# Autodesk Inventor part: Kettenrad der Rollenkette1
Saved by Autodesk Inventor 2016 (Build 200138000, 138)
## iProperties
Created: 2017-12-11
Part Number: Kettenrad der Rollenkette1
Material: Steel
Document SubType Name: Modeling
Designer: Dominik
Density: 1 g/cm^3
Appearance: Steel
CustomPartVersion: 1
Author: Dominik
Autodesk Inventor part; units mm, degrees
ref_plane "YZ Plane" through (0, 0, 0) normal (1, 0, 0) x (0, 1, 0)
ref_plane "XZ Plane" through (0, 0, 0) normal (0, 1, 0) x (-1, 0, 0)
sketch "Theoretisches Zahnprofil" plane through (0, 0, 0) normal (0, 0, 1) x (1, 0, 0)
  circle A0 centre (0, 0) radius 24.3021 construction
  line L0 (0, 0) -> (0, 24.3021) construction
  line L1 (0, 0) -> (7.8909, 22.9854) construction
  circle A1 centre (0, 0) radius 26.3707
  arc A2 (-1.9854, 22.7421) -> (1.9854, 22.7421) centre (0, 24.3021) ccw
  line L2 (0, 24.3021) -> (7.8909, 22.9854) construction
  line L3 (0, 24.3021) -> (3.1452, 26.7735) construction
  line L4 (3.1452, 26.7735) -> (-2.8564, 24.2129) construction
  arc A3 (3.9692, 26.0703) -> (3.0961, 24.7748) centre (6.9045, 23.15) ccw
  arc A4 (-3.0961, 24.7748) -> (-3.9692, 26.0703) centre (-6.9045, 23.15) ccw
  line L5 (-6.9045, 23.15) -> (-3.0961, 24.7748) construction
  arc A5 (-2.8564, 24.2129) -> (-1.9854, 22.7421) centre (3.1452, 26.7735) ccw
  line L6 (-2.8564, 24.2129) -> (-3.0961, 24.7748)
  arc A6 (1.9854, 22.7421) -> (2.8564, 24.2129) centre (-3.1452, 26.7735) ccw
  line L7 (3.0961, 24.7748) -> (2.8564, 24.2129)
  line L8 (0, 0) -> (4.3405, 26.011) construction
  point P0 (3.9454, 23.6438)
  dimension "d0" = 48.6043
  dimension "d2" = 18.947
  dimension "d3" = 2.525
  dimension "d10" = 128.158
  dimension "d11" = 15.053
  dimension "d12" = 4
  dimension "d13" = 6.525
  dimension "d14" = 7
  dimension "d23" = 2.4
  constraints: 18 end point, 15 point on circle, 7 centre point, 3 coincident, 3 point on line, 3 symmetric about line, 3 tangent, 1 equal radius, 1 midpoint, 1 parallel, 1 vertical, 1 other
  measures "d0" diameter of A0
  measures "d2" angle of L1 L0
  measures "d3" radius of A2
  measures "d10" angle of L3 L0
  measures "d11" angle of L4 L3
  measures "d12" distance of L2.start L3.end
  measures "d13" distance of L3.end L4.end
  measures "d14" distance of A3.centre L0.end
  measures "d23" distance from line of L8.end L2
sketch "Zahnprofil" plane through (0, 0, 0) normal (0, 0, 1) x (1, 0, 0)
  arc A0 (-2.335, 23.3412) -> (2.335, 23.3412) centre (0, 24.3021) ccw
  arc A1 (3.8891, 26.0823) -> (2.335, 23.3412) centre (13.9869, 18.5462) ccw
  arc A2 (-2.335, 23.3412) -> (-3.8891, 26.0823) centre (-13.9869, 18.5462) ccw
  line L0 (0, 0) -> (0, 24.3021) construction
  line L1 (0, 24.3021) -> (2.335, 23.3412) construction
  line L2 (0, 24.3021) -> (-2.335, 23.3412) construction
  circle A3 centre (0, 0) radius 26.3707 projected
  dimension "d44" = 135.263
  dimension "d45" = 12.6
  dimension "d46" = 2.525
  constraints: 9 point on circle, 6 end point, 3 centre point, 2 tangent, 1 coincident, 1 equal radius, 1 vertical, 1 other
  measures "d44" angle of L2 L1
  measures "d45" radius of A1
  measures "d46" radius of A0
sketch "Schnittprofil" plane through (0, 0, 0) normal (1, 0, 0) x (0, 1, 0)
  line L0 (26.3707, 0) -> (-26.3707, 0) projected
  line L1 (16.1535, 1.395) -> (-16.1535, 1.395)
  line L2 (-16.1535, 1.395) -> (-16.1535, -1.395)
  line L3 (-16.1535, -1.395) -> (16.1535, -1.395)
  line L4 (16.1535, -1.395) -> (16.1535, 1.395)
  line L5 (16.1535, 1.395) -> (26.3707, 1.395) construction
  line L6 (26.3707, 1.395) -> (26.3707, -1.395) construction
  line L7 (26.3707, -1.395) -> (16.1535, -1.395) construction
  line L8 (16.1535, -1.395) -> (16.1535, 1.395)
  arc A0 (26.3707, 0.355) -> (22.4263, 1.395) centre (22.4263, -6.605) ccw
  arc A1 (22.4263, -1.395) -> (26.3707, -0.355) centre (22.4263, 6.605) ccw
  line L9 (22.4263, 1.395) -> (0, 1.395)
  line L10 (0, 1.395) -> (0, -1.395)
  line L11 (0, -1.395) -> (22.4263, -1.395)
  line L12 (0, 1.395) -> (0, -1.395)
  line L13 (26.3707, 0.355) -> (26.3707, -0.355)
  point P0 (0, 0)
  point P1 (0, 0)
  dimension "d30" = 2.79
  dimension "d31" = 32.307
  dimension "d32" = 2.79
  dimension "d33" = 1.04
  dimension "d34" = 8
  dimension "d43" = 1.395
  constraints: 26 end point, 7 midpoint, 5 perpendicular, 4 parallel, 4 point on circle, 3 point on line, 3 symmetric about line, 2 centre point, 2 horizontal, 2 tangent, 1 collinear, 1 other
  measures "d30" distance between parallel lines of L7 L5
  measures "d31" distance between parallel lines of L2 L4
  measures "d32" distance between parallel lines of L3 L1
  measures "d33" distance from line of L13.start L5
  measures "d34" radius of A0
  measures "d43" distance between parallel lines of L3 L0
revolve "Ummantelung" add sketch "Schnittprofil" angle 360 about axis through (0, 0, 1.395) along (0, 0, -1) contours L10 L3 L2 L0 | L0 L2 L1 L10
revolve "Reihe" add sketch "Schnittprofil" angle 360 about axis through (0, 0, 1.395) along (0, 0, -1) contours L13 A1 L11 L4 L0 | L0 L4 L9 A0 L13 | L4 L3 L10 L0 | L0 L10 L1 L4
pattern_of_one "Reihenanordnung"
extrude "Theoretischer Zahn" cut sketch "Theoretisches Zahnprofil" along normal through all both and the other way through all contours A3 L7 A6 A2 A5 L6 A4 A1 picked at (0, 24.8172)
extrude "Zahn" [suppressed]
pattern_circular "Zahnanordnung" count 19 over 360 about axis through (0, 0, -10) along (0, 0, 1) of "Theoretischer Zahn"
ref_plane "Planungsebene" through (0, 24.3021, 0) normal (1, 0, 0) x (0, 1, 0)
equation "\"d3\" = 0.5 * da_Dr + da_SC"
equation "\"d12\" = 0.8 * da_Dr"
equation "\"d13\" = 1.3 * da_Dr + da_SC"
equation "\"d14\" = 1.4 * da_Dr"
equation "\"d23\" = da_Ha"
equation "\"d44\" = da_Alfa"
equation "\"d45\" = da_Re"
equation "\"d46\" = da_Ri"
equation "\"d30\" = da_Bf"
equation "\"d31\" = da_Ds"
equation "\"d32\" = da_Bs"
equation "\"d33\" = da_Ba"
equation "\"d34\" = da_Rx"
equation "\"d40\" = da_pt"
equation "\"form_type\" = 0"
equation "\"da_p\" = 8"
equation "\"da_Dr\" = 5"
equation "\"da_SC\" = 0.025"
equation "\"da_Ha\" = 2.4"
equation "\"da_pt\" = 5.64"
equation "\"da_Bf\" = 2.79"
equation "\"da_Ba\" = 1.04"
equation "\"da_Rx\" = 8"
equation "\"da_Ra\" = 0.32"
equation "\"da_Bs\" = 2.79"
equation "\"da_Ds\" = 32.30697"
equation "\"da_Re\" = 12.6"
equation "\"da_Ri\" = 2.525"
equation "\"da_Alfa\" = 135.263deg"
body "Solid1"
